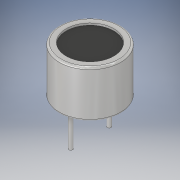
# Autodesk Inventor part: Ultraschallwandler16mm
Saved by Autodesk Inventor 2019 (Build 230136000, 136)
## iProperties
Created: 2018-08-21
Part Number: Ultraschallwandler16mm
Material: Generisch
Document SubType Name: Modeling
Designer: Sven
Density: 1 g/cm^3
Appearance: Vorgabe
Author: Sven
Autodesk Inventor part; units mm, degrees
ref_plane "YZ Plane" through (0, 0, 0) normal (1, 0, 0) x (0, 1, 0)
ref_plane "XZ Plane" through (0, 0, 0) normal (0, 1, 0) x (-1, 0, 0)
ref_plane "XY Plane" through (0, 0, 0) normal (0, 0, 1) x (1, 0, 0)
sketch "Skizze1" plane through (0, 0, 0) normal (0, 1, 0) x (-1, 0, 0)
  circle A0 centre (0, 0) radius 8
  dimension "d0" = 16
  constraints: 1 centre point, 1 coincident
  measures "d0" diameter of A0
extrude "Extrusion1" add sketch "Skizze1" along normal blind 12.2
fillet "Rundung1" radius 0.5 2 edges at (8, 12.2, 0) (8, 0, 0)
sketch "Skizze2" plane through (0, 12.2, 0) normal (0, 1, 0) x (1, 0, 0)
  circle A0 centre (0, 0) radius 6.2
  circle A1 centre (0, 0) radius 8 projected
  dimension "d4" = 1.8
  constraints: 1 centre point, 1 coincident
  measures "d4" radial gap between concentric circles of A0 A1
extrude "Extrusion2" cut sketch "Skizze2" against normal blind 0.5 contours A0
sketch "Skizze3" plane through (0, 0, 0) normal (0, -1, 0) x (1, 0, 0)
  circle A0 centre (0, 0) radius 7.5
  constraints: 1 centre point, 1 coincident
extrude "Extrusion3" cut sketch "Skizze3" against normal blind 0.75
sketch "Skizze4" plane through (0, 0.75, 0) normal (0, -1, 0) x (1, 0, 0)
  circle A0 centre (0, -5) radius 0.5
  circle A1 centre (0, 5) radius 0.5
  point P0 (0, 0)
  dimension "d9" = 10
  dimension "d10" = 5
  dimension "d11" = 1
  dimension "d12" = 1
  constraints: 2 centre point
  measures "d9" distance of A1.centre A0.centre
  measures "d10" distance of point (0, 0) A0.centre
  measures "d11" diameter of A1
  measures "d12" diameter of A0
extrude "Extrusion4" add sketch "Skizze4" along normal blind 10
sketch "Skizze5" plane through (0, 0.75, 0) normal (0, -1, 0) x (1, 0, 0)
  circle A0 centre (0, -5) radius 0.5
  circle A1 centre (0, -5) radius 1.5
  circle A2 centre (0, 5) radius 0.5
  circle A3 centre (0, 5) radius 0.75
  circle A4 centre (0, 5) radius 0.5 projected
  circle A5 centre (0, -5) radius 0.5 projected
  point P0 (0, 0)
  dimension "d15" = 0
  dimension "d16" = 0
  dimension "d17" = 1
  dimension "d18" = 0.25
  constraints: 4 centre point, 2 coincident, 2 concentric
  measures "d15" radial gap between concentric circles of A4 A2
  measures "d16" radial gap between concentric circles of A5 A0
  measures "d17" radial gap between concentric circles of A0 A1
  measures "d18" radial gap between concentric circles of A2 A3
extrude "Extrusion5" cut sketch "Skizze5" against normal blind 0.1
equation "\"d10\" = 0.5 * d9"
equation "\"d12\" = d11"
